cable holder 2 (Autodesk Fusion 360 design; units mm, degrees)
Autodesk Fusion 360 part; units mm, degrees
note: some values were not read from the file. Set by a fixed rule: which sketch regions a step uses.
sketch "Sketch1" plane through (0, 0, 0) normal (0, 1, 0) x (1, 0, 0)
  line L0 (0, 0) -> (6, 0)
  line L1 (6, 0) -> (6, -1.5)
  line L2 (6, -1.5) -> (0, -1.5)
  line L3 (0, -1.5) -> (0, 0)
  line L4 (6, 0) -> (7.5, 0)
  line L5 (7.5, 0) -> (7.5, -4)
  line L6 (7.5, -4) -> (6, -4)
  line L7 (6, -4) -> (6, 0)
  line L8 (6, -4) -> (20, -4)
  line L9 (20, -4) -> (20, -5.5)
  line L10 (20, -5.5) -> (6, -5.5)
  line L11 (6, -5.5) -> (6, -4)
  line L12 (20, -4) -> (18.5, -4)
  line L13 (18.5, -4) -> (18.5, 0)
  line L14 (18.5, 0) -> (20, 0)
  line L15 (20, 0) -> (20, -4)
  line L16 (20, 0) -> (26, 0)
  line L17 (26, 0) -> (26, -1.5)
  line L18 (26, -1.5) -> (20, -1.5)
  line L19 (20, -1.5) -> (20, 0)
  dimension "d1" = 6
  dimension "d2" = 1.5
  dimension "d3" = 1.5
  dimension "d4" = 4
  dimension "d5" = 14
  dimension "d6" = 1.5
  dimension "d7" = 1.5
  dimension "d8" = 4
  dimension "d9" = 6
  dimension "d10" = 1.5
  constraint horizontal L0
  constraint vertical L1
  constraint horizontal L2
  constraint vertical L3
  constraint coincident L0.start L3.end
  constraint horizontal L4
  constraint vertical L5
  constraint horizontal L6
  constraint vertical L7
  constraint horizontal L8
  constraint vertical L9
  constraint horizontal L10
  constraint vertical L11
  constraint horizontal L12
  constraint vertical L13
  constraint horizontal L14
  constraint vertical L15
  constraint horizontal L16
  constraint vertical L17
  constraint horizontal L18
  constraint vertical L19
  measures "d1" distance of L0.start L0.end
  measures "d2" distance of L0.start L2.end
  measures "d3" distance of L0.end L4.end
  measures "d4" distance of L0.end L6.end
  measures "d5" distance of L6.end L8.end
  measures "d6" distance of L6.end L10.end
  measures "d7" distance of L8.end L12.end
  measures "d8" distance of L8.end L14.end
  measures "d9" distance of L14.end L16.end
  measures "d10" distance of L14.end L18.end
extrude "Extrude1" add sketch "Sketch1" along normal blind 8
sketch "Sketch2" plane through (0, 0, 1.5) normal (0, 0, 1) x (-1, 0, 0)
  line L0 (0, 0) -> (-6, 0)
  line L1 (-6, 0) -> (-6, -8)
  line L2 (-6, -8) -> (0, -8)
  line L3 (0, -8) -> (0, 0)
  line L4 (0, -8) -> (-6, 0)
  line L5 (-20, -8) -> (-26, 0)
  circle A0 centre (-3, -4) radius 1
  circle A1 centre (-23, -4) radius 1
  point P0 (-3, -4)
  point P1 (-23, -4)
  point P2 (-26, 0)
  point P3 (-20, -8)
  dimension "d13" = 2
  dimension "d14" = 2
  constraint coincident L2.end L3.start
  constraint coincident L0.end L1.start
  constraint midpoint L4 P0
  constraint midpoint L5 P1
  constraint coincident P0 A0.centre
  constraint coincident P1 A1.centre
  constraint coincident P2 L5.end
  constraint coincident P3 L5.start
  measures "d13" diameter of A0
  measures "d14" diameter of A1
extrude "Extrude2" cut sketch "Sketch2" against normal blind 2 contours L4 A0 | L4 A0 | L5 A1 | L5 A1
sketch "Sketch3" plane through (0, 0, 0) normal (0, 1, 0) x (1, 0, 0)
